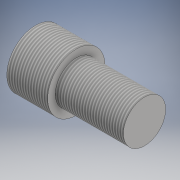
# Autodesk Inventor part: nuts
Saved by Autodesk Inventor 2017 (Build 210142000, 142)
## iProperties
Created: 2018-02-22
Part Number: nuts
Material: Generic
Document SubType Name: Modeling
Designer: CMRU-CAD-PC 11
Density: 1 g/cm^3
Appearance: Default
Author: CMRU-CAD-PC 11
Autodesk Inventor part; units mm, degrees
ref_plane "YZ Plane" through (0, 0, 0) normal (1, 0, 0) x (0, 1, 0)
ref_plane "XZ Plane" through (0, 0, 0) normal (0, 1, 0) x (-1, 0, 0)
ref_plane "XY Plane" through (0, 0, 0) normal (0, 0, 1) x (1, 0, 0)
sketch "Sketch1" plane through (0, 0, 0) normal (1, 0, 0) x (0, 1, 0)
  circle A0 centre (0, 0) radius 7.7505
  constraints: 1 centre point, 1 coincident
extrude "Extrusion1" add sketch "Sketch1" along normal blind 25
thread "Thread1" size "M10x1" class "6g" standard "ANSI Metric M Profile" full length
sketch "Sketch2" plane through (0, 0, 0) normal (-1, 0, 0) x (0, 0, 1)
  point P0 (0, 0)
sketch "Sketch3" plane through (0, 0, 0) normal (-1, 0, 0) x (0, 0, 1)
  circle A0 centre (0, 0) radius 10.5233
  line L0 (5.6968, -4.4416) -> (-0.9981, -7.1543)
  line L1 (-0.9981, -7.1543) -> (-6.6949, -2.7128)
  line L2 (-6.6949, -2.7128) -> (-5.6968, 4.4416)
  line L3 (-5.6968, 4.4416) -> (0.9981, 7.1543)
  line L4 (0.9981, 7.1543) -> (6.6949, 2.7128)
  line L5 (6.6949, 2.7128) -> (5.6968, -4.4416)
  constraints: 12 end point, 2 coincident, 1 centre point, 13 other
extrude "Extrusion2" add sketch "Sketch3" along normal blind 15
sketch "Sketch4" plane through (0, 0, 0) normal (-1, 0, 0) x (0, 0, 1)
  point P0 (0, 0)
sketch "Sketch5" plane through (0, 0, 0) normal (-1, 0, 0) x (0, 0, 1)
  point P0 (0, 0)
thread "Thread2" size "M10x1" class "6g" standard "ANSI Metric M Profile" full length
body "Solid1"
